Autodesk Fusion 360 part; units mm, degrees
note: some values were not read from the file. Chosen so that the rebuilt part matches the saved one: which face or edge a step refers to. Set by a fixed rule: which sketch regions a step uses.
(part 3 of 3)
sketch "Hex Side" plane through (0, 0, 0) normal (1, 0, 0) x (0, 1, 0)
  line L0 (0, 0) -> (-0.001, 0) construction
  line L1 (-0.001, 0) -> (-0.001, 1) construction
  line L2 (-0.001, 1) -> (0, 1) construction
  line L3 (0, 1) -> (0, 0) construction
  line L4 (-1.9518, 4.3789) -> (-3.9026, 1)
  line L5 (-3.9026, 1) -> (-1.9518, -2.3789)
  line L6 (-1.9518, -2.3789) -> (1.9498, -2.3789)
  line L7 (1.9498, -2.3789) -> (3.9006, 1)
  line L8 (3.9006, 1) -> (1.9498, 4.3789)
  line L9 (1.9498, 4.3789) -> (-1.9518, 4.3789)
  line L10 (-0.001, 1) -> (2.9252, 2.6894) construction
  line L11 (-0.001, 1) -> (-0.001, -2.3789) construction
  line L12 (4.9396, 8.3576) -> (2.9888, 4.9787)
  line L13 (8.8412, 8.3576) -> (4.9396, 8.3576)
  line L14 (2.9888, 4.9787) -> (4.9396, 1.5999)
  line L15 (4.9396, 1.5999) -> (8.8412, 1.5999)
  line L16 (8.8412, 1.5999) -> (10.792, 4.9787)
  line L17 (10.792, 4.9787) -> (8.8412, 8.3576)
  line L18 (2.9252, 2.6894) -> (3.9644, 3.2894)
  line L19 (-61.6828, -7.5574) -> (-65.5844, -7.5574)
  line L20 (-65.5844, -7.5574) -> (-67.5352, -10.9363)
  line L21 (-59.732, -10.9363) -> (-61.6828, -7.5574)
  line L22 (-61.6828, -14.3151) -> (-59.732, -10.9363)
  line L23 (-65.5844, -14.3151) -> (-61.6828, -14.3151)
  line L24 (-67.5352, -10.9363) -> (-65.5844, -14.3151)
  line L25 (-66.6234, -14.915) -> (-68.5742, -11.5361)
  line L26 (-68.5742, -18.2939) -> (-66.6234, -14.915)
  line L27 (-72.4758, -18.2939) -> (-68.5742, -18.2939)
  line L28 (-68.5742, -11.5361) -> (-72.4758, -11.5361)
  line L29 (-72.4758, -11.5361) -> (-74.4266, -14.915)
  line L30 (-74.4266, -14.915) -> (-72.4758, -18.2939)
  line L31 (-47.578, 0.4001) -> (-51.4796, 0.4001)
  line L32 (-51.4796, 0.4001) -> (-53.4304, -2.9788)
  line L33 (-45.6272, -2.9788) -> (-47.578, 0.4001)
  line L34 (-47.578, -6.3576) -> (-45.6272, -2.9788)
  line L35 (-51.4796, -6.3576) -> (-47.578, -6.3576)
  line L36 (-53.4304, -2.9788) -> (-51.4796, -6.3576)
  line L37 (-52.5186, -6.9575) -> (-54.4694, -3.5786)
  line L38 (-54.4694, -10.3364) -> (-52.5186, -6.9575)
  line L39 (-58.371, -10.3364) -> (-54.4694, -10.3364)
  line L40 (-54.4694, -3.5786) -> (-58.371, -3.5786)
  line L41 (-58.371, -3.5786) -> (-60.3218, -6.9575)
  line L42 (-60.3218, -6.9575) -> (-58.371, -10.3364)
  line L43 (-0.001, 4.3789) -> (-0.001, 5.5789)
  line L44 (3.9006, 1) -> (9.0022, 1) construction
  line L45 (9.0022, 1) -> (9.0022, -0.4851) construction
  line L46 (-47.578, -7.5574) -> (-51.4796, -7.5574)
  line L47 (-51.4796, -7.5574) -> (-53.4304, -10.9363)
  line L48 (-45.6272, -10.9363) -> (-47.578, -7.5574)
  line L49 (-47.578, -14.3151) -> (-45.6272, -10.9363)
  line L50 (-51.4796, -14.3151) -> (-47.578, -14.3151)
  line L51 (-53.4304, -10.9363) -> (-51.4796, -14.3151)
  line L52 (-52.5186, -14.915) -> (-54.4694, -11.5361)
  line L53 (-54.4694, -18.2939) -> (-52.5186, -14.915)
  line L54 (-58.371, -18.2939) -> (-54.4694, -18.2939)
  line L55 (-54.4694, -11.5361) -> (-58.371, -11.5361)
  line L56 (-58.371, -11.5361) -> (-60.3218, -14.915)
  line L57 (-60.3218, -14.915) -> (-58.371, -18.2939)
  line L58 (-61.6828, 0.4001) -> (-65.5844, 0.4001)
  line L59 (-65.5844, 0.4001) -> (-67.5352, -2.9788)
  line L60 (-59.732, -2.9788) -> (-61.6828, 0.4001)
  line L61 (-61.6828, -6.3576) -> (-59.732, -2.9788)
  line L62 (-65.5844, -6.3576) -> (-61.6828, -6.3576)
  line L63 (-67.5352, -2.9788) -> (-65.5844, -6.3576)
  line L64 (-66.6234, -6.9575) -> (-68.5742, -3.5786)
  line L65 (-68.5742, -10.3364) -> (-66.6234, -6.9575)
  line L66 (-72.4758, -10.3364) -> (-68.5742, -10.3364)
  line L67 (-68.5742, -3.5786) -> (-72.4758, -3.5786)
  line L68 (-72.4758, -3.5786) -> (-74.4266, -6.9575)
  line L69 (-74.4266, -6.9575) -> (-72.4758, -10.3364)
  line L70 (-61.6828, 8.3576) -> (-65.5844, 8.3576)
  line L71 (-65.5844, 8.3576) -> (-67.5352, 4.9787)
  line L72 (-59.732, 4.9787) -> (-61.6828, 8.3576)
  line L73 (-61.6828, 1.5999) -> (-59.732, 4.9787)
  line L74 (-65.5844, 1.5999) -> (-61.6828, 1.5999)
  line L75 (-67.5352, 4.9787) -> (-65.5844, 1.5999)
  line L76 (-66.6234, 1) -> (-68.5742, 4.3789)
  line L77 (-68.5742, -2.3789) -> (-66.6234, 1)
  line L78 (-72.4758, -2.3789) -> (-68.5742, -2.3789)
  line L79 (-68.5742, 4.3789) -> (-72.4758, 4.3789)
  line L80 (-72.4758, 4.3789) -> (-74.4266, 1)
  line L81 (-74.4266, 1) -> (-72.4758, -2.3789)
  line L82 (9.0022, 1) -> (10.2022, 1) construction
  line L83 (-33.4732, -7.5574) -> (-37.3748, -7.5574)
  line L84 (-37.3748, -7.5574) -> (-39.3256, -10.9363)
  line L85 (-31.5224, -10.9363) -> (-33.4732, -7.5574)
  line L86 (-33.4732, -14.3151) -> (-31.5224, -10.9363)
  line L87 (-37.3748, -14.3151) -> (-33.4732, -14.3151)
  line L88 (-39.3256, -10.9363) -> (-37.3748, -14.3151)
  line L89 (-38.4138, -14.915) -> (-40.3646, -11.5361)
  line L90 (-40.3646, -18.2939) -> (-38.4138, -14.915)
  line L91 (-44.2662, -18.2939) -> (-40.3646, -18.2939)
  line L92 (-40.3646, -11.5361) -> (-44.2662, -11.5361)
  line L93 (-44.2662, -11.5361) -> (-46.217, -14.915)
  line L94 (-46.217, -14.915) -> (-44.2662, -18.2939)
  line L95 (-19.3684, -7.5574) -> (-23.27, -7.5574)
  line L96 (-23.27, -7.5574) -> (-25.2208, -10.9363)
  line L97 (-17.4176, -10.9363) -> (-19.3684, -7.5574)
  line L98 (-19.3684, -14.3151) -> (-17.4176, -10.9363)
  line L99 (-23.27, -14.3151) -> (-19.3684, -14.3151)
  line L100 (-25.2208, -10.9363) -> (-23.27, -14.3151)
  line L101 (-24.309, -14.915) -> (-26.2598, -11.5361)
  line L102 (-26.2598, -18.2939) -> (-24.309, -14.915)
  line L103 (-30.1614, -18.2939) -> (-26.2598, -18.2939)
  line L104 (-26.2598, -11.5361) -> (-30.1614, -11.5361)
  line L105 (-30.1614, -11.5361) -> (-32.1122, -14.915)
  line L106 (-32.1122, -14.915) -> (-30.1614, -18.2939)
  line L107 (-5.2636, -7.5574) -> (-9.1652, -7.5574)
  line L108 (-9.1652, -7.5574) -> (-11.116, -10.9363)
  line L109 (-3.3128, -10.9363) -> (-5.2636, -7.5574)
  line L110 (-5.2636, -14.3151) -> (-3.3128, -10.9363)
  line L111 (-9.1652, -14.3151) -> (-5.2636, -14.3151)
  line L112 (-11.116, -10.9363) -> (-9.1652, -14.3151)
  line L113 (-10.2042, -14.915) -> (-12.155, -11.5361)
  line L114 (-12.155, -18.2939) -> (-10.2042, -14.915)
  line L115 (-16.0566, -18.2939) -> (-12.155, -18.2939)
  line L116 (-12.155, -11.5361) -> (-16.0566, -11.5361)
  line L117 (-16.0566, -11.5361) -> (-18.0074, -14.915)
  line L118 (-18.0074, -14.915) -> (-16.0566, -18.2939)
  line L119 (8.8412, -7.5574) -> (4.9396, -7.5574)
  line L120 (4.9396, -7.5574) -> (2.9888, -10.9363)
  line L121 (10.792, -10.9363) -> (8.8412, -7.5574)
  line L122 (8.8412, -14.3151) -> (10.792, -10.9363)
  line L123 (4.9396, -14.3151) -> (8.8412, -14.3151)
  line L124 (2.9888, -10.9363) -> (4.9396, -14.3151)
  line L125 (3.9006, -14.915) -> (1.9498, -11.5361)
  line L126 (1.9498, -18.2939) -> (3.9006, -14.915)
  line L127 (-1.9518, -18.2939) -> (1.9498, -18.2939)
  line L128 (1.9498, -11.5361) -> (-1.9518, -11.5361)
  line L129 (-1.9518, -11.5361) -> (-3.9026, -14.915)
  line L130 (-3.9026, -14.915) -> (-1.9518, -18.2939)
  line L131 (22.946, -7.5574) -> (19.0444, -7.5574)
  line L132 (19.0444, -7.5574) -> (17.0936, -10.9363)
  line L133 (24.8968, -10.9363) -> (22.946, -7.5574)
  line L134 (22.946, -14.3151) -> (24.8968, -10.9363)
  line L135 (19.0444, -14.3151) -> (22.946, -14.3151)
  line L136 (17.0936, -10.9363) -> (19.0444, -14.3151)
  line L137 (18.0054, -14.915) -> (16.0546, -11.5361)
  line L138 (16.0546, -18.2939) -> (18.0054, -14.915)
  line L139 (12.153, -18.2939) -> (16.0546, -18.2939)
  line L140 (16.0546, -11.5361) -> (12.153, -11.5361)
  line L141 (12.153, -11.5361) -> (10.2022, -14.915)
  line L142 (10.2022, -14.915) -> (12.153, -18.2939)
  line L143 (37.0508, -7.5574) -> (33.1492, -7.5574)
  line L144 (33.1492, -7.5574) -> (31.1984, -10.9363)
  line L145 (39.0016, -10.9363) -> (37.0508, -7.5574)
  line L146 (37.0508, -14.3151) -> (39.0016, -10.9363)
  line L147 (33.1492, -14.3151) -> (37.0508, -14.3151)
  line L148 (31.1984, -10.9363) -> (33.1492, -14.3151)
  line L149 (32.1102, -14.915) -> (30.1594, -11.5361)
  line L150 (30.1594, -18.2939) -> (32.1102, -14.915)
  line L151 (26.2578, -18.2939) -> (30.1594, -18.2939)
  line L152 (30.1594, -11.5361) -> (26.2578, -11.5361)
  line L153 (26.2578, -11.5361) -> (24.307, -14.915)
  line L154 (24.307, -14.915) -> (26.2578, -18.2939)
  line L155 (51.1556, -7.5574) -> (47.254, -7.5574)
  line L156 (47.254, -7.5574) -> (45.3032, -10.9363)
  line L157 (53.1064, -10.9363) -> (51.1556, -7.5574)
  line L158 (51.1556, -14.3151) -> (53.1064, -10.9363)
  line L159 (47.254, -14.3151) -> (51.1556, -14.3151)
  line L160 (45.3032, -10.9363) -> (47.254, -14.3151)
  line L161 (46.215, -14.915) -> (44.2642, -11.5361)
  line L162 (44.2642, -18.2939) -> (46.215, -14.915)
  line L163 (40.3626, -18.2939) -> (44.2642, -18.2939)
  line L164 (44.2642, -11.5361) -> (40.3626, -11.5361)
  line L165 (40.3626, -11.5361) -> (38.4118, -14.915)
  line L166 (38.4118, -14.915) -> (40.3626, -18.2939)
  line L167 (65.2604, -7.5574) -> (61.3588, -7.5574)
  line L168 (61.3588, -7.5574) -> (59.408, -10.9363)
  line L169 (67.2112, -10.9363) -> (65.2604, -7.5574)
  line L170 (65.2604, -14.3151) -> (67.2112, -10.9363)
  line L171 (61.3588, -14.3151) -> (65.2604, -14.3151)
  line L172 (59.408, -10.9363) -> (61.3588, -14.3151)
  line L173 (60.3198, -14.915) -> (58.369, -11.5361)
  line L174 (58.369, -18.2939) -> (60.3198, -14.915)
  line L175 (54.4674, -18.2939) -> (58.369, -18.2939)
  line L176 (58.369, -11.5361) -> (54.4674, -11.5361)
  line L177 (54.4674, -11.5361) -> (52.5166, -14.915)
  line L178 (52.5166, -14.915) -> (54.4674, -18.2939)
  line L179 (79.3652, -7.5574) -> (75.4636, -7.5574)
  line L180 (75.4636, -7.5574) -> (73.5128, -10.9363)
  line L181 (81.316, -10.9363) -> (79.3652, -7.5574)
  line L182 (79.3652, -14.3151) -> (81.316, -10.9363)
  line L183 (75.4636, -14.3151) -> (79.3652, -14.3151)
  line L184 (73.5128, -10.9363) -> (75.4636, -14.3151)
  line L185 (74.4246, -14.915) -> (72.4738, -11.5361)
  line L186 (72.4738, -18.2939) -> (74.4246, -14.915)
  line L187 (68.5722, -18.2939) -> (72.4738, -18.2939)
  line L188 (72.4738, -11.5361) -> (68.5722, -11.5361)
  line L189 (68.5722, -11.5361) -> (66.6214, -14.915)
  line L190 (66.6214, -14.915) -> (68.5722, -18.2939)
  line L191 (-33.4732, 0.4001) -> (-37.3748, 0.4001)
  line L192 (-37.3748, 0.4001) -> (-39.3256, -2.9788)
  line L193 (-31.5224, -2.9788) -> (-33.4732, 0.4001)
  line L194 (-33.4732, -6.3576) -> (-31.5224, -2.9788)
  line L195 (-37.3748, -6.3576) -> (-33.4732, -6.3576)
  line L196 (-39.3256, -2.9788) -> (-37.3748, -6.3576)
  line L197 (-38.4138, -6.9575) -> (-40.3646, -3.5786)
  line L198 (-40.3646, -10.3364) -> (-38.4138, -6.9575)
  line L199 (-44.2662, -10.3364) -> (-40.3646, -10.3364)
  line L200 (-40.3646, -3.5786) -> (-44.2662, -3.5786)
  line L201 (-44.2662, -3.5786) -> (-46.217, -6.9575)
  line L202 (-46.217, -6.9575) -> (-44.2662, -10.3364)
  line L203 (-19.3684, 0.4001) -> (-23.27, 0.4001)
  line L204 (-23.27, 0.4001) -> (-25.2208, -2.9788)
  line L205 (-17.4176, -2.9788) -> (-19.3684, 0.4001)
  line L206 (-19.3684, -6.3576) -> (-17.4176, -2.9788)
  line L207 (-23.27, -6.3576) -> (-19.3684, -6.3576)
  line L208 (-25.2208, -2.9788) -> (-23.27, -6.3576)
  line L209 (-24.309, -6.9575) -> (-26.2598, -3.5786)
  line L210 (-26.2598, -10.3364) -> (-24.309, -6.9575)
  line L211 (-30.1614, -10.3364) -> (-26.2598, -10.3364)
  line L212 (-26.2598, -3.5786) -> (-30.1614, -3.5786)
  line L213 (-30.1614, -3.5786) -> (-32.1122, -6.9575)
  line L214 (-32.1122, -6.9575) -> (-30.1614, -10.3364)
  line L215 (-5.2636, 0.4001) -> (-9.1652, 0.4001)
  line L216 (-9.1652, 0.4001) -> (-11.116, -2.9788)
  line L217 (-3.3128, -2.9788) -> (-5.2636, 0.4001)
  line L218 (-5.2636, -6.3576) -> (-3.3128, -2.9788)
  line L219 (-9.1652, -6.3576) -> (-5.2636, -6.3576)
  line L220 (-11.116, -2.9788) -> (-9.1652, -6.3576)
  line L221 (-10.2042, -6.9575) -> (-12.155, -3.5786)
  line L222 (-12.155, -10.3364) -> (-10.2042, -6.9575)
  line L223 (-16.0566, -10.3364) -> (-12.155, -10.3364)
  line L224 (-12.155, -3.5786) -> (-16.0566, -3.5786)
  line L225 (-16.0566, -3.5786) -> (-18.0074, -6.9575)
  line L226 (-18.0074, -6.9575) -> (-16.0566, -10.3364)
  line L227 (8.8412, 0.4001) -> (4.9396, 0.4001)
  line L228 (4.9396, 0.4001) -> (2.9888, -2.9788)
  line L229 (10.792, -2.9788) -> (8.8412, 0.4001)
  line L230 (8.8412, -6.3576) -> (10.792, -2.9788)
  line L231 (4.9396, -6.3576) -> (8.8412, -6.3576)
  line L232 (2.9888, -2.9788) -> (4.9396, -6.3576)
  line L233 (3.9006, -6.9575) -> (1.9498, -3.5786)
  line L234 (1.9498, -10.3364) -> (3.9006, -6.9575)
  line L235 (-1.9518, -10.3364) -> (1.9498, -10.3364)
  line L236 (1.9498, -3.5786) -> (-1.9518, -3.5786)
  line L237 (-1.9518, -3.5786) -> (-3.9026, -6.9575)
  line L238 (-3.9026, -6.9575) -> (-1.9518, -10.3364)
  line L239 (22.946, 0.4001) -> (19.0444, 0.4001)
  line L240 (19.0444, 0.4001) -> (17.0936, -2.9788)
  line L241 (24.8968, -2.9788) -> (22.946, 0.4001)
  line L242 (22.946, -6.3576) -> (24.8968, -2.9788)
  line L243 (19.0444, -6.3576) -> (22.946, -6.3576)
  line L244 (17.0936, -2.9788) -> (19.0444, -6.3576)
  line L245 (18.0054, -6.9575) -> (16.0546, -3.5786)
  line L246 (16.0546, -10.3364) -> (18.0054, -6.9575)
  line L247 (12.153, -10.3364) -> (16.0546, -10.3364)
  line L248 (16.0546, -3.5786) -> (12.153, -3.5786)
  line L249 (12.153, -3.5786) -> (10.2022, -6.9575)
  line L250 (10.2022, -6.9575) -> (12.153, -10.3364)
  line L251 (37.0508, 0.4001) -> (33.1492, 0.4001)
  line L252 (33.1492, 0.4001) -> (31.1984, -2.9788)
  line L253 (39.0016, -2.9788) -> (37.0508, 0.4001)
  line L254 (37.0508, -6.3576) -> (39.0016, -2.9788)
  line L255 (33.1492, -6.3576) -> (37.0508, -6.3576)
  line L256 (31.1984, -2.9788) -> (33.1492, -6.3576)
  line L257 (32.1102, -6.9575) -> (30.1594, -3.5786)
  line L258 (30.1594, -10.3364) -> (32.1102, -6.9575)
  line L259 (26.2578, -10.3364) -> (30.1594, -10.3364)
  line L260 (30.1594, -3.5786) -> (26.2578, -3.5786)
  line L261 (26.2578, -3.5786) -> (24.307, -6.9575)
  line L262 (24.307, -6.9575) -> (26.2578, -10.3364)
  line L263 (51.1556, 0.4001) -> (47.254, 0.4001)
  line L264 (47.254, 0.4001) -> (45.3032, -2.9788)
  line L265 (53.1064, -2.9788) -> (51.1556, 0.4001)
  line L266 (51.1556, -6.3576) -> (53.1064, -2.9788)
  line L267 (47.254, -6.3576) -> (51.1556, -6.3576)
  line L268 (45.3032, -2.9788) -> (47.254, -6.3576)
  line L269 (46.215, -6.9575) -> (44.2642, -3.5786)
  line L270 (44.2642, -10.3364) -> (46.215, -6.9575)
  line L271 (40.3626, -10.3364) -> (44.2642, -10.3364)
  line L272 (44.2642, -3.5786) -> (40.3626, -3.5786)
  line L273 (40.3626, -3.5786) -> (38.4118, -6.9575)
  line L274 (38.4118, -6.9575) -> (40.3626, -10.3364)
  line L275 (65.2604, 0.4001) -> (61.3588, 0.4001)
  line L276 (61.3588, 0.4001) -> (59.408, -2.9788)
  line L277 (67.2112, -2.9788) -> (65.2604, 0.4001)
  line L278 (65.2604, -6.3576) -> (67.2112, -2.9788)
  line L279 (61.3588, -6.3576) -> (65.2604, -6.3576)
  line L280 (59.408, -2.9788) -> (61.3588, -6.3576)
  line L281 (60.3198, -6.9575) -> (58.369, -3.5786)
  line L282 (58.369, -10.3364) -> (60.3198, -6.9575)
  line L283 (54.4674, -10.3364) -> (58.369, -10.3364)
  line L284 (58.369, -3.5786) -> (54.4674, -3.5786)
  line L285 (54.4674, -3.5786) -> (52.5166, -6.9575)
  line L286 (52.5166, -6.9575) -> (54.4674, -10.3364)
  line L287 (79.3652, 0.4001) -> (75.4636, 0.4001)
  line L288 (75.4636, 0.4001) -> (73.5128, -2.9788)
  line L289 (81.316, -2.9788) -> (79.3652, 0.4001)
  line L290 (79.3652, -6.3576) -> (81.316, -2.9788)
  line L291 (75.4636, -6.3576) -> (79.3652, -6.3576)
  line L292 (73.5128, -2.9788) -> (75.4636, -6.3576)
  line L293 (74.4246, -6.9575) -> (72.4738, -3.5786)
  line L294 (72.4738, -10.3364) -> (74.4246, -6.9575)
  line L295 (68.5722, -10.3364) -> (72.4738, -10.3364)
  line L296 (72.4738, -3.5786) -> (68.5722, -3.5786)
  line L297 (68.5722, -3.5786) -> (66.6214, -6.9575)
  line L298 (66.6214, -6.9575) -> (68.5722, -10.3364)
  line L299 (-47.578, 8.3576) -> (-51.4796, 8.3576)
  line L300 (-51.4796, 8.3576) -> (-53.4304, 4.9787)
  line L301 (-45.6272, 4.9787) -> (-47.578, 8.3576)
  line L302 (-47.578, 1.5999) -> (-45.6272, 4.9787)
  line L303 (-51.4796, 1.5999) -> (-47.578, 1.5999)
  line L304 (-53.4304, 4.9787) -> (-51.4796, 1.5999)
  line L305 (-52.5186, 1) -> (-54.4694, 4.3789)
  line L306 (-54.4694, -2.3789) -> (-52.5186, 1)
  line L307 (-58.371, -2.3789) -> (-54.4694, -2.3789)
  line L308 (-54.4694, 4.3789) -> (-58.371, 4.3789)
  line L309 (-58.371, 4.3789) -> (-60.3218, 1)
  line L310 (-60.3218, 1) -> (-58.371, -2.3789)
  line L311 (-33.4732, 8.3576) -> (-37.3748, 8.3576)
  line L312 (-37.3748, 8.3576) -> (-39.3256, 4.9787)
  line L313 (-31.5224, 4.9787) -> (-33.4732, 8.3576)
  line L314 (-33.4732, 1.5999) -> (-31.5224, 4.9787)
  line L315 (-37.3748, 1.5999) -> (-33.4732, 1.5999)
  line L316 (-39.3256, 4.9787) -> (-37.3748, 1.5999)
  line L317 (-38.4138, 1) -> (-40.3646, 4.3789)
  line L318 (-40.3646, -2.3789) -> (-38.4138, 1)
  line L319 (-44.2662, -2.3789) -> (-40.3646, -2.3789)
  line L320 (-40.3646, 4.3789) -> (-44.2662, 4.3789)
  line L321 (-44.2662, 4.3789) -> (-46.217, 1)
  line L322 (-46.217, 1) -> (-44.2662, -2.3789)
  line L323 (-19.3684, 8.3576) -> (-23.27, 8.3576)
  line L324 (-23.27, 8.3576) -> (-25.2208, 4.9787)
  line L325 (-17.4176, 4.9787) -> (-19.3684, 8.3576)
  line L326 (-19.3684, 1.5999) -> (-17.4176, 4.9787)
  line L327 (-23.27, 1.5999) -> (-19.3684, 1.5999)
  line L328 (-25.2208, 4.9787) -> (-23.27, 1.5999)
  line L329 (-24.309, 1) -> (-26.2598, 4.3789)
  line L330 (-26.2598, -2.3789) -> (-24.309, 1)
  line L331 (-30.1614, -2.3789) -> (-26.2598, -2.3789)
  line L332 (-26.2598, 4.3789) -> (-30.1614, 4.3789)
  line L333 (-30.1614, 4.3789) -> (-32.1122, 1)
  line L334 (-32.1122, 1) -> (-30.1614, -2.3789)
  line L335 (-5.2636, 8.3576) -> (-9.1652, 8.3576)
  line L336 (-9.1652, 8.3576) -> (-11.116, 4.9787)
  line L337 (-3.3128, 4.9787) -> (-5.2636, 8.3576)
  line L338 (-5.2636, 1.5999) -> (-3.3128, 4.9787)
  line L339 (-9.1652, 1.5999) -> (-5.2636, 1.5999)
  line L340 (-11.116, 4.9787) -> (-9.1652, 1.5999)
  line L341 (-10.2042, 1) -> (-12.155, 4.3789)
  line L342 (-12.155, -2.3789) -> (-10.2042, 1)
  line L343 (-16.0566, -2.3789) -> (-12.155, -2.3789)
  line L344 (-12.155, 4.3789) -> (-16.0566, 4.3789)
  line L345 (-16.0566, 4.3789) -> (-18.0074, 1)
  line L346 (-18.0074, 1) -> (-16.0566, -2.3789)
  line L347 (22.946, 8.3576) -> (19.0444, 8.3576)
  line L348 (19.0444, 8.3576) -> (17.0936, 4.9787)
  line L349 (24.8968, 4.9787) -> (22.946, 8.3576)
  line L350 (22.946, 1.5999) -> (24.8968, 4.9787)
  line L351 (19.0444, 1.5999) -> (22.946, 1.5999)
  line L352 (17.0936, 4.9787) -> (19.0444, 1.5999)
  line L353 (18.0054, 1) -> (16.0546, 4.3789)
  line L354 (16.0546, -2.3789) -> (18.0054, 1)
  line L355 (12.153, -2.3789) -> (16.0546, -2.3789)
  line L356 (16.0546, 4.3789) -> (12.153, 4.3789)
  line L357 (12.153, 4.3789) -> (10.2022, 1)
  line L358 (10.2022, 1) -> (12.153, -2.3789)
  line L359 (37.0508, 8.3576) -> (33.1492, 8.3576)
  line L360 (33.1492, 8.3576) -> (31.1984, 4.9787)
  line L361 (39.0016, 4.9787) -> (37.0508, 8.3576)
  line L362 (37.0508, 1.5999) -> (39.0016, 4.9787)
  line L363 (33.1492, 1.5999) -> (37.0508, 1.5999)
  line L364 (31.1984, 4.9787) -> (33.1492, 1.5999)
  line L365 (32.1102, 1) -> (30.1594, 4.3789)
  line L366 (30.1594, -2.3789) -> (32.1102, 1)
  line L367 (26.2578, -2.3789) -> (30.1594, -2.3789)
  line L368 (30.1594, 4.3789) -> (26.2578, 4.3789)
  line L369 (26.2578, 4.3789) -> (24.307, 1)
  line L370 (24.307, 1) -> (26.2578, -2.3789)
  line L371 (51.1556, 8.3576) -> (47.254, 8.3576)
  line L372 (47.254, 8.3576) -> (45.3032, 4.9787)
  line L373 (53.1064, 4.9787) -> (51.1556, 8.3576)
  line L374 (51.1556, 1.5999) -> (53.1064, 4.9787)
  line L375 (47.254, 1.5999) -> (51.1556, 1.5999)
  line L376 (45.3032, 4.9787) -> (47.254, 1.5999)
  line L377 (46.215, 1) -> (44.2642, 4.3789)
  line L378 (44.2642, -2.3789) -> (46.215, 1)
  line L379 (40.3626, -2.3789) -> (44.2642, -2.3789)
  line L380 (44.2642, 4.3789) -> (40.3626, 4.3789)
  line L381 (40.3626, 4.3789) -> (38.4118, 1)
  line L382 (38.4118, 1) -> (40.3626, -2.3789)
  line L383 (65.2604, 8.3576) -> (61.3588, 8.3576)
  line L384 (61.3588, 8.3576) -> (59.408, 4.9787)
  line L385 (67.2112, 4.9787) -> (65.2604, 8.3576)
  line L386 (65.2604, 1.5999) -> (67.2112, 4.9787)
  line L387 (61.3588, 1.5999) -> (65.2604, 1.5999)
  line L388 (59.408, 4.9787) -> (61.3588, 1.5999)
  line L389 (60.3198, 1) -> (58.369, 4.3789)
  line L390 (58.369, -2.3789) -> (60.3198, 1)
  line L391 (54.4674, -2.3789) -> (58.369, -2.3789)
  line L392 (58.369, 4.3789) -> (54.4674, 4.3789)
  line L393 (54.4674, 4.3789) -> (52.5166, 1)
  line L394 (52.5166, 1) -> (54.4674, -2.3789)
  line L395 (79.3652, 8.3576) -> (75.4636, 8.3576)
  line L396 (75.4636, 8.3576) -> (73.5128, 4.9787)
  line L397 (81.316, 4.9787) -> (79.3652, 8.3576)
  line L398 (79.3652, 1.5999) -> (81.316, 4.9787)
  line L399 (75.4636, 1.5999) -> (79.3652, 1.5999)
  line L400 (73.5128, 4.9787) -> (75.4636, 1.5999)
  line L401 (74.4246, 1) -> (72.4738, 4.3789)
  line L402 (72.4738, -2.3789) -> (74.4246, 1)
  line L403 (68.5722, -2.3789) -> (72.4738, -2.3789)
  line L404 (72.4738, 4.3789) -> (68.5722, 4.3789)
  line L405 (68.5722, 4.3789) -> (66.6214, 1)
  line L406 (66.6214, 1) -> (68.5722, -2.3789)
  line L407 (-61.6828, 16.3151) -> (-65.5844, 16.3151)
  line L408 (-65.5844, 16.3151) -> (-67.5352, 12.9362)
  line L409 (-59.732, 12.9362) -> (-61.6828, 16.3151)
  line L410 (-61.6828, 9.5574) -> (-59.732, 12.9362)
  line L411 (-65.5844, 9.5574) -> (-61.6828, 9.5574)
  line L412 (-67.5352, 12.9362) -> (-65.5844, 9.5574)
  line L413 (-66.6234, 8.9575) -> (-68.5742, 12.3364)
  line L414 (-68.5742, 5.5786) -> (-66.6234, 8.9575)
  line L415 (-72.4758, 5.5786) -> (-68.5742, 5.5786)
  line L416 (-68.5742, 12.3364) -> (-72.4758, 12.3364)
  line L417 (-72.4758, 12.3364) -> (-74.4266, 8.9575)
  line L418 (-74.4266, 8.9575) -> (-72.4758, 5.5786)
  line L419 (-47.578, 16.3151) -> (-51.4796, 16.3151)
  line L420 (-51.4796, 16.3151) -> (-53.4304, 12.9362)
  line L421 (-45.6272, 12.9362) -> (-47.578, 16.3151)
  line L422 (-47.578, 9.5574) -> (-45.6272, 12.9362)
  line L423 (-51.4796, 9.5574) -> (-47.578, 9.5574)
  line L424 (-53.4304, 12.9362) -> (-51.4796, 9.5574)
  line L425 (-52.5186, 8.9575) -> (-54.4694, 12.3364)
  line L426 (-54.4694, 5.5786) -> (-52.5186, 8.9575)
  line L427 (-58.371, 5.5786) -> (-54.4694, 5.5786)
  line L428 (-54.4694, 12.3364) -> (-58.371, 12.3364)
  line L429 (-58.371, 12.3364) -> (-60.3218, 8.9575)
  line L430 (-60.3218, 8.9575) -> (-58.371, 5.5786)
  line L431 (-33.4732, 16.3151) -> (-37.3748, 16.3151)
  line L432 (-37.3748, 16.3151) -> (-39.3256, 12.9362)
  line L433 (-31.5224, 12.9362) -> (-33.4732, 16.3151)
  line L434 (-33.4732, 9.5574) -> (-31.5224, 12.9362)
  line L435 (-37.3748, 9.5574) -> (-33.4732, 9.5574)
  line L436 (-39.3256, 12.9362) -> (-37.3748, 9.5574)
  line L437 (-38.4138, 8.9575) -> (-40.3646, 12.3364)
  line L438 (-40.3646, 5.5786) -> (-38.4138, 8.9575)
  line L439 (-44.2662, 5.5786) -> (-40.3646, 5.5786)
  line L440 (-40.3646, 12.3364) -> (-44.2662, 12.3364)
  line L441 (-44.2662, 12.3364) -> (-46.217, 8.9575)
  line L442 (-46.217, 8.9575) -> (-44.2662, 5.5786)
  line L443 (-19.3684, 16.3151) -> (-23.27, 16.3151)
  line L444 (-23.27, 16.3151) -> (-25.2208, 12.9362)
  line L445 (-17.4176, 12.9362) -> (-19.3684, 16.3151)
  line L446 (-19.3684, 9.5574) -> (-17.4176, 12.9362)
  line L447 (-23.27, 9.5574) -> (-19.3684, 9.5574)
  line L448 (-25.2208, 12.9362) -> (-23.27, 9.5574)
  line L449 (-24.309, 8.9575) -> (-26.2598, 12.3364)
  line L450 (-26.2598, 5.5786) -> (-24.309, 8.9575)
  line L451 (-30.1614, 5.5786) -> (-26.2598, 5.5786)
  line L452 (-26.2598, 12.3364) -> (-30.1614, 12.3364)
  line L453 (-30.1614, 12.3364) -> (-32.1122, 8.9575)
  line L454 (-32.1122, 8.9575) -> (-30.1614, 5.5786)
  line L455 (-5.2636, 16.3151) -> (-9.1652, 16.3151)
  line L456 (-9.1652, 16.3151) -> (-11.116, 12.9362)
  line L457 (-3.3128, 12.9362) -> (-5.2636, 16.3151)
  line L458 (-5.2636, 9.5574) -> (-3.3128, 12.9362)
  line L459 (-9.1652, 9.5574) -> (-5.2636, 9.5574)
  line L460 (-11.116, 12.9362) -> (-9.1652, 9.5574)
  line L461 (-10.2042, 8.9575) -> (-12.155, 12.3364)
  line L462 (-12.155, 5.5786) -> (-10.2042, 8.9575)
  line L463 (-16.0566, 5.5786) -> (-12.155, 5.5786)
  line L464 (-12.155, 12.3364) -> (-16.0566, 12.3364)
  line L465 (-16.0566, 12.3364) -> (-18.0074, 8.9575)
  line L466 (-18.0074, 8.9575) -> (-16.0566, 5.5786)
  line L467 (8.8412, 16.3151) -> (4.9396, 16.3151)
  line L468 (4.9396, 16.3151) -> (2.9888, 12.9362)
  line L469 (10.792, 12.9362) -> (8.8412, 16.3151)
  line L470 (8.8412, 9.5574) -> (10.792, 12.9362)
  line L471 (4.9396, 9.5574) -> (8.8412, 9.5574)
  line L472 (2.9888, 12.9362) -> (4.9396, 9.5574)
  line L473 (3.9006, 8.9575) -> (1.9498, 12.3364)
  line L474 (1.9498, 5.5786) -> (3.9006, 8.9575)
  line L475 (-1.9518, 5.5786) -> (1.9498, 5.5786)
  line L476 (1.9498, 12.3364) -> (-1.9518, 12.3364)
  line L477 (-1.9518, 12.3364) -> (-3.9026, 8.9575)
  line L478 (-3.9026, 8.9575) -> (-1.9518, 5.5786)
  line L479 (22.946, 16.3151) -> (19.0444, 16.3151)
  line L480 (19.0444, 16.3151) -> (17.0936, 12.9362)
  line L481 (24.8968, 12.9362) -> (22.946, 16.3151)
  line L482 (22.946, 9.5574) -> (24.8968, 12.9362)
  line L483 (19.0444, 9.5574) -> (22.946, 9.5574)
  line L484 (17.0936, 12.9362) -> (19.0444, 9.5574)
  line L485 (18.0054, 8.9575) -> (16.0546, 12.3364)
  line L486 (16.0546, 5.5786) -> (18.0054, 8.9575)
  line L487 (12.153, 5.5786) -> (16.0546, 5.5786)
  line L488 (16.0546, 12.3364) -> (12.153, 12.3364)
  line L489 (12.153, 12.3364) -> (10.2022, 8.9575)
  line L490 (10.2022, 8.9575) -> (12.153, 5.5786)
  line L491 (37.0508, 16.3151) -> (33.1492, 16.3151)
  line L492 (33.1492, 16.3151) -> (31.1984, 12.9362)
  line L493 (39.0016, 12.9362) -> (37.0508, 16.3151)
  line L494 (37.0508, 9.5574) -> (39.0016, 12.9362)
  line L495 (33.1492, 9.5574) -> (37.0508, 9.5574)
  line L496 (31.1984, 12.9362) -> (33.1492, 9.5574)
  line L497 (32.1102, 8.9575) -> (30.1594, 12.3364)
  line L498 (30.1594, 5.5786) -> (32.1102, 8.9575)
  line L499 (26.2578, 5.5786) -> (30.1594, 5.5786)
  line L500 (30.1594, 12.3364) -> (26.2578, 12.3364)
  line L501 (26.2578, 12.3364) -> (24.307, 8.9575)
  line L502 (24.307, 8.9575) -> (26.2578, 5.5786)
  line L503 (51.1556, 16.3151) -> (47.254, 16.3151)
  line L504 (47.254, 16.3151) -> (45.3032, 12.9362)
  line L505 (53.1064, 12.9362) -> (51.1556, 16.3151)
  line L506 (51.1556, 9.5574) -> (53.1064, 12.9362)
  line L507 (47.254, 9.5574) -> (51.1556, 9.5574)
  line L508 (45.3032, 12.9362) -> (47.254, 9.5574)
  line L509 (46.215, 8.9575) -> (44.2642, 12.3364)
  line L510 (44.2642, 5.5786) -> (46.215, 8.9575)
  line L511 (40.3626, 5.5786) -> (44.2642, 5.5786)
  line L512 (44.2642, 12.3364) -> (40.3626, 12.3364)
  line L513 (40.3626, 12.3364) -> (38.4118, 8.9575)
  line L514 (38.4118, 8.9575) -> (40.3626, 5.5786)
  line L515 (65.2604, 16.3151) -> (61.3588, 16.3151)
  line L516 (61.3588, 16.3151) -> (59.408, 12.9362)
  line L517 (67.2112, 12.9362) -> (65.2604, 16.3151)
  line L518 (65.2604, 9.5574) -> (67.2112, 12.9362)
  line L519 (61.3588, 9.5574) -> (65.2604, 9.5574)
  line L520 (59.408, 12.9362) -> (61.3588, 9.5574)
  line L521 (60.3198, 8.9575) -> (58.369, 12.3364)
  line L522 (58.369, 5.5786) -> (60.3198, 8.9575)
  line L523 (54.4674, 5.5786) -> (58.369, 5.5786)
  line L524 (58.369, 12.3364) -> (54.4674, 12.3364)
  line L525 (54.4674, 12.3364) -> (52.5166, 8.9575)
  line L526 (52.5166, 8.9575) -> (54.4674, 5.5786)
  line L527 (79.3652, 16.3151) -> (75.4636, 16.3151)
  line L528 (75.4636, 16.3151) -> (73.5128, 12.9362)
  line L529 (81.316, 12.9362) -> (79.3652, 16.3151)
  line L530 (79.3652, 9.5574) -> (81.316, 12.9362)
  line L531 (75.4636, 9.5574) -> (79.3652, 9.5574)
  line L532 (73.5128, 12.9362) -> (75.4636, 9.5574)
  line L533 (74.4246, 8.9575) -> (72.4738, 12.3364)
  line L534 (72.4738, 5.5786) -> (74.4246, 8.9575)
  line L535 (68.5722, 5.5786) -> (72.4738, 5.5786)
  line L536 (72.4738, 12.3364) -> (68.5722, 12.3364)
  line L537 (68.5722, 12.3364) -> (66.6214, 8.9575)
  line L538 (66.6214, 8.9575) -> (68.5722, 5.5786)
  line L539 (-61.6828, 24.2726) -> (-65.5844, 24.2726)
  line L540 (-65.5844, 24.2726) -> (-67.5352, 20.8937)
  line L541 (-59.732, 20.8937) -> (-61.6828, 24.2726)
  line L542 (-61.6828, 17.5149) -> (-59.732, 20.8937)
  line L543 (-65.5844, 17.5149) -> (-61.6828, 17.5149)
  line L544 (-67.5352, 20.8937) -> (-65.5844, 17.5149)
  line L545 (-66.6234, 16.915) -> (-68.5742, 20.2939)
  line L546 (-68.5742, 13.5361) -> (-66.6234, 16.915)
  line L547 (-72.4758, 13.5361) -> (-68.5742, 13.5361)
  line L548 (-68.5742, 20.2939) -> (-72.4758, 20.2939)
  line L549 (-72.4758, 20.2939) -> (-74.4266, 16.915)
  line L550 (-74.4266, 16.915) -> (-72.4758, 13.5361)
  line L551 (-47.578, 24.2726) -> (-51.4796, 24.2726)
  line L552 (-51.4796, 24.2726) -> (-53.4304, 20.8937)
  line L553 (-45.6272, 20.8937) -> (-47.578, 24.2726)
  line L554 (-47.578, 17.5149) -> (-45.6272, 20.8937)
  line L555 (-51.4796, 17.5149) -> (-47.578, 17.5149)
  line L556 (-53.4304, 20.8937) -> (-51.4796, 17.5149)
  line L557 (-52.5186, 16.915) -> (-54.4694, 20.2939)
  line L558 (-54.4694, 13.5361) -> (-52.5186, 16.915)
  line L559 (-58.371, 13.5361) -> (-54.4694, 13.5361)
  line L560 (-54.4694, 20.2939) -> (-58.371, 20.2939)
  line L561 (-58.371, 20.2939) -> (-60.3218, 16.915)
  line L562 (-60.3218, 16.915) -> (-58.371, 13.5361)
  line L563 (-33.4732, 24.2726) -> (-37.3748, 24.2726)
  line L564 (-37.3748, 24.2726) -> (-39.3256, 20.8937)
  line L565 (-31.5224, 20.8937) -> (-33.4732, 24.2726)
  line L566 (-33.4732, 17.5149) -> (-31.5224, 20.8937)
  line L567 (-37.3748, 17.5149) -> (-33.4732, 17.5149)
  line L568 (-39.3256, 20.8937) -> (-37.3748, 17.5149)
  line L569 (-38.4138, 16.915) -> (-40.3646, 20.2939)
  line L570 (-40.3646, 13.5361) -> (-38.4138, 16.915)
  line L571 (-44.2662, 13.5361) -> (-40.3646, 13.5361)
  line L572 (-40.3646, 20.2939) -> (-44.2662, 20.2939)
  line L573 (-44.2662, 20.2939) -> (-46.217, 16.915)
  line L574 (-46.217, 16.915) -> (-44.2662, 13.5361)
  line L575 (-19.3684, 24.2726) -> (-23.27, 24.2726)
  line L576 (-23.27, 24.2726) -> (-25.2208, 20.8937)
  line L577 (-17.4176, 20.8937) -> (-19.3684, 24.2726)
  line L578 (-19.3684, 17.5149) -> (-17.4176, 20.8937)
  line L579 (-23.27, 17.5149) -> (-19.3684, 17.5149)
  line L580 (-25.2208, 20.8937) -> (-23.27, 17.5149)
  line L581 (-24.309, 16.915) -> (-26.2598, 20.2939)
  line L582 (-26.2598, 13.5361) -> (-24.309, 16.915)
  line L583 (-30.1614, 13.5361) -> (-26.2598, 13.5361)
  line L584 (-26.2598, 20.2939) -> (-30.1614, 20.2939)
  line L585 (-30.1614, 20.2939) -> (-32.1122, 16.915)
  line L586 (-32.1122, 16.915) -> (-30.1614, 13.5361)
  line L587 (-5.2636, 24.2726) -> (-9.1652, 24.2726)
  line L588 (-9.1652, 24.2726) -> (-11.116, 20.8937)
  line L589 (-3.3128, 20.8937) -> (-5.2636, 24.2726)
  line L590 (-5.2636, 17.5149) -> (-3.3128, 20.8937)
  line L591 (-9.1652, 17.5149) -> (-5.2636, 17.5149)
  line L592 (-11.116, 20.8937) -> (-9.1652, 17.5149)
  line L593 (-10.2042, 16.915) -> (-12.155, 20.2939)
  line L594 (-12.155, 13.5361) -> (-10.2042, 16.915)
  line L595 (-16.0566, 13.5361) -> (-12.155, 13.5361)
  line L596 (-12.155, 20.2939) -> (-16.0566, 20.2939)
  line L597 (-16.0566, 20.2939) -> (-18.0074, 16.915)
  line L598 (-18.0074, 16.915) -> (-16.0566, 13.5361)
  line L599 (8.8412, 24.2726) -> (4.9396, 24.2726)
  line L600 (4.9396, 24.2726) -> (2.9888, 20.8937)
  line L601 (10.792, 20.8937) -> (8.8412, 24.2726)
  line L602 (8.8412, 17.5149) -> (10.792, 20.8937)
  line L603 (4.9396, 17.5149) -> (8.8412, 17.5149)
  line L604 (2.9888, 20.8937) -> (4.9396, 17.5149)
  line L605 (3.9006, 16.915) -> (1.9498, 20.2939)
  line L606 (1.9498, 13.5361) -> (3.9006, 16.915)
  line L607 (-1.9518, 13.5361) -> (1.9498, 13.5361)
  line L608 (1.9498, 20.2939) -> (-1.9518, 20.2939)
  line L609 (-1.9518, 20.2939) -> (-3.9026, 16.915)
  line L610 (-3.9026, 16.915) -> (-1.9518, 13.5361)
  line L611 (22.946, 24.2726) -> (19.0444, 24.2726)
  line L612 (19.0444, 24.2726) -> (17.0936, 20.8937)
  line L613 (24.8968, 20.8937) -> (22.946, 24.2726)
  line L614 (22.946, 17.5149) -> (24.8968, 20.8937)
  line L615 (19.0444, 17.5149) -> (22.946, 17.5149)
  line L616 (17.0936, 20.8937) -> (19.0444, 17.5149)
  line L617 (18.0054, 16.915) -> (16.0546, 20.2939)
  line L618 (16.0546, 13.5361) -> (18.0054, 16.915)
  line L619 (12.153, 13.5361) -> (16.0546, 13.5361)
  line L620 (16.0546, 20.2939) -> (12.153, 20.2939)
  line L621 (12.153, 20.2939) -> (10.2022, 16.915)
  line L622 (10.2022, 16.915) -> (12.153, 13.5361)
  line L623 (37.0508, 24.2726) -> (33.1492, 24.2726)
  line L624 (33.1492, 24.2726) -> (31.1984, 20.8937)
  line L625 (39.0016, 20.8937) -> (37.0508, 24.2726)
  line L626 (37.0508, 17.5149) -> (39.0016, 20.8937)
  line L627 (33.1492, 17.5149) -> (37.0508, 17.5149)
  line L628 (31.1984, 20.8937) -> (33.1492, 17.5149)
  line L629 (32.1102, 16.915) -> (30.1594, 20.2939)
  line L630 (30.1594, 13.5361) -> (32.1102, 16.915)
  line L631 (26.2578, 13.5361) -> (30.1594, 13.5361)
  line L632 (30.1594, 20.2939) -> (26.2578, 20.2939)
  line L633 (26.2578, 20.2939) -> (24.307, 16.915)
  line L634 (24.307, 16.915) -> (26.2578, 13.5361)
  line L635 (51.1556, 24.2726) -> (47.254, 24.2726)
  line L636 (47.254, 24.2726) -> (45.3032, 20.8937)
  line L637 (53.1064, 20.8937) -> (51.1556, 24.2726)
  line L638 (51.1556, 17.5149) -> (53.1064, 20.8937)
  line L639 (47.254, 17.5149) -> (51.1556, 17.5149)
  line L640 (45.3032, 20.8937) -> (47.254, 17.5149)
  line L641 (46.215, 16.915) -> (44.2642, 20.2939)
  line L642 (44.2642, 13.5361) -> (46.215, 16.915)
  line L643 (40.3626, 13.5361) -> (44.2642, 13.5361)
  line L644 (44.2642, 20.2939) -> (40.3626, 20.2939)
  line L645 (40.3626, 20.2939) -> (38.4118, 16.915)
  line L646 (38.4118, 16.915) -> (40.3626, 13.5361)
  line L647 (65.2604, 24.2726) -> (61.3588, 24.2726)
  line L648 (61.3588, 24.2726) -> (59.408, 20.8937)
  line L649 (67.2112, 20.8937) -> (65.2604, 24.2726)
  line L650 (65.2604, 17.5149) -> (67.2112, 20.8937)
  line L651 (61.3588, 17.5149) -> (65.2604, 17.5149)
  line L652 (59.408, 20.8937) -> (61.3588, 17.5149)
  line L653 (60.3198, 16.915) -> (58.369, 20.2939)
  line L654 (58.369, 13.5361) -> (60.3198, 16.915)
  line L655 (54.4674, 13.5361) -> (58.369, 13.5361)
  line L656 (58.369, 20.2939) -> (54.4674, 20.2939)
  line L657 (54.4674, 20.2939) -> (52.5166, 16.915)
  line L658 (52.5166, 16.915) -> (54.4674, 13.5361)
  line L659 (79.3652, 24.2726) -> (75.4636, 24.2726)
  line L660 (75.4636, 24.2726) -> (73.5128, 20.8937)
  line L661 (81.316, 20.8937) -> (79.3652, 24.2726)
  line L662 (79.3652, 17.5149) -> (81.316, 20.8937)
  line L663 (75.4636, 17.5149) -> (79.3652, 17.5149)
  line L664 (73.5128, 20.8937) -> (75.4636, 17.5149)
  line L665 (74.4246, 16.915) -> (72.4738, 20.2939)
  line L666 (72.4738, 13.5361) -> (74.4246, 16.915)
  line L667 (68.5722, 13.5361) -> (72.4738, 13.5361)
  line L668 (72.4738, 20.2939) -> (68.5722, 20.2939)
  line L669 (68.5722, 20.2939) -> (66.6214, 16.915)
  line L670 (66.6214, 16.915) -> (68.5722, 13.5361)
  line L671 (-61.6828, 32.2301) -> (-65.5844, 32.2301)
  line L672 (-65.5844, 32.2301) -> (-67.5352, 28.8512)
  line L673 (-59.732, 28.8512) -> (-61.6828, 32.2301)
  line L674 (-61.6828, 25.4724) -> (-59.732, 28.8512)
  line L675 (-65.5844, 25.4724) -> (-61.6828, 25.4724)
  line L676 (-67.5352, 28.8512) -> (-65.5844, 25.4724)
  line L677 (-66.6234, 24.8725) -> (-68.5742, 28.2514)
  line L678 (-68.5742, 21.4936) -> (-66.6234, 24.8725)
  line L679 (-72.4758, 21.4936) -> (-68.5742, 21.4936)
  line L680 (-68.5742, 28.2514) -> (-72.4758, 28.2514)
  line L681 (-72.4758, 28.2514) -> (-74.4266, 24.8725)
  line L682 (-74.4266, 24.8725) -> (-72.4758, 21.4936)
  line L683 (-47.578, 32.2301) -> (-51.4796, 32.2301)
  line L684 (-51.4796, 32.2301) -> (-53.4304, 28.8512)
  line L685 (-45.6272, 28.8512) -> (-47.578, 32.2301)
  line L686 (-47.578, 25.4724) -> (-45.6272, 28.8512)
  line L687 (-51.4796, 25.4724) -> (-47.578, 25.4724)
  line L688 (-53.4304, 28.8512) -> (-51.4796, 25.4724)
  line L689 (-52.5186, 24.8725) -> (-54.4694, 28.2514)
  line L690 (-54.4694, 21.4936) -> (-52.5186, 24.8725)
  line L691 (-58.371, 21.4936) -> (-54.4694, 21.4936)
  line L692 (-54.4694, 28.2514) -> (-58.371, 28.2514)
  line L693 (-58.371, 28.2514) -> (-60.3218, 24.8725)
  line L694 (-60.3218, 24.8725) -> (-58.371, 21.4936)
  line L695 (-33.4732, 32.2301) -> (-37.3748, 32.2301)
  line L696 (-37.3748, 32.2301) -> (-39.3256, 28.8512)
  line L697 (-31.5224, 28.8512) -> (-33.4732, 32.2301)
  line L698 (-33.4732, 25.4724) -> (-31.5224, 28.8512)
  line L699 (-37.3748, 25.4724) -> (-33.4732, 25.4724)
  line L700 (-39.3256, 28.8512) -> (-37.3748, 25.4724)
  line L701 (-38.4138, 24.8725) -> (-40.3646, 28.2514)
  line L702 (-40.3646, 21.4936) -> (-38.4138, 24.8725)
  line L703 (-44.2662, 21.4936) -> (-40.3646, 21.4936)
  line L704 (-40.3646, 28.2514) -> (-44.2662, 28.2514)
  line L705 (-44.2662, 28.2514) -> (-46.217, 24.8725)
  line L706 (-46.217, 24.8725) -> (-44.2662, 21.4936)
  line L707 (-19.3684, 32.2301) -> (-23.27, 32.2301)
  line L708 (-23.27, 32.2301) -> (-25.2208, 28.8512)
  line L709 (-17.4176, 28.8512) -> (-19.3684, 32.2301)
  line L710 (-19.3684, 25.4724) -> (-17.4176, 28.8512)
  line L711 (-23.27, 25.4724) -> (-19.3684, 25.4724)
  line L712 (-25.2208, 28.8512) -> (-23.27, 25.4724)
  line L713 (-24.309, 24.8725) -> (-26.2598, 28.2514)
  line L714 (-26.2598, 21.4936) -> (-24.309, 24.8725)
  line L715 (-30.1614, 21.4936) -> (-26.2598, 21.4936)
  line L716 (-26.2598, 28.2514) -> (-30.1614, 28.2514)
  line L717 (-30.1614, 28.2514) -> (-32.1122, 24.8725)
  line L718 (-32.1122, 24.8725) -> (-30.1614, 21.4936)
  line L719 (-5.2636, 32.2301) -> (-9.1652, 32.2301)
  line L720 (-9.1652, 32.2301) -> (-11.116, 28.8512)
  line L721 (-3.3128, 28.8512) -> (-5.2636, 32.2301)
  line L722 (-5.2636, 25.4724) -> (-3.3128, 28.8512)
  line L723 (-9.1652, 25.4724) -> (-5.2636, 25.4724)
  line L724 (-11.116, 28.8512) -> (-9.1652, 25.4724)
  line L725 (-10.2042, 24.8725) -> (-12.155, 28.2514)
  line L726 (-12.155, 21.4936) -> (-10.2042, 24.8725)
  line L727 (-16.0566, 21.4936) -> (-12.155, 21.4936)
  line L728 (-12.155, 28.2514) -> (-16.0566, 28.2514)
  line L729 (-16.0566, 28.2514) -> (-18.0074, 24.8725)
  line L730 (-18.0074, 24.8725) -> (-16.0566, 21.4936)
  line L731 (8.8412, 32.2301) -> (4.9396, 32.2301)
  line L732 (4.9396, 32.2301) -> (2.9888, 28.8512)
  line L733 (10.792, 28.8512) -> (8.8412, 32.2301)
  line L734 (8.8412, 25.4724) -> (10.792, 28.8512)
  line L735 (4.9396, 25.4724) -> (8.8412, 25.4724)
  line L736 (2.9888, 28.8512) -> (4.9396, 25.4724)
  line L737 (3.9006, 24.8725) -> (1.9498, 28.2514)
  line L738 (1.9498, 21.4936) -> (3.9006, 24.8725)
  line L739 (-1.9518, 21.4936) -> (1.9498, 21.4936)
  line L740 (1.9498, 28.2514) -> (-1.9518, 28.2514)
  line L741 (-1.9518, 28.2514) -> (-3.9026, 24.8725)
  line L742 (-3.9026, 24.8725) -> (-1.9518, 21.4936)
  line L743 (22.946, 32.2301) -> (19.0444, 32.2301)
  line L744 (19.0444, 32.2301) -> (17.0936, 28.8512)
  line L745 (24.8968, 28.8512) -> (22.946, 32.2301)
  line L746 (22.946, 25.4724) -> (24.8968, 28.8512)
  line L747 (19.0444, 25.4724) -> (22.946, 25.4724)
  line L748 (17.0936, 28.8512) -> (19.0444, 25.4724)
  line L749 (18.0054, 24.8725) -> (16.0546, 28.2514)
  line L750 (16.0546, 21.4936) -> (18.0054, 24.8725)
  line L751 (12.153, 21.4936) -> (16.0546, 21.4936)
  line L752 (16.0546, 28.2514) -> (12.153, 28.2514)
  line L753 (12.153, 28.2514) -> (10.2022, 24.8725)
  line L754 (10.2022, 24.8725) -> (12.153, 21.4936)
  line L755 (37.0508, 32.2301) -> (33.1492, 32.2301)
  line L756 (33.1492, 32.2301) -> (31.1984, 28.8512)
  line L757 (39.0016, 28.8512) -> (37.0508, 32.2301)
  line L758 (37.0508, 25.4724) -> (39.0016, 28.8512)
  line L759 (33.1492, 25.4724) -> (37.0508, 25.4724)
  line L760 (31.1984, 28.8512) -> (33.1492, 25.4724)
  line L761 (32.1102, 24.8725) -> (30.1594, 28.2514)
  line L762 (30.1594, 21.4936) -> (32.1102, 24.8725)
  line L763 (26.2578, 21.4936) -> (30.1594, 21.4936)
  line L764 (30.1594, 28.2514) -> (26.2578, 28.2514)
  line L765 (26.2578, 28.2514) -> (24.307, 24.8725)
  line L766 (24.307, 24.8725) -> (26.2578, 21.4936)
  line L767 (51.1556, 32.2301) -> (47.254, 32.2301)
  line L768 (47.254, 32.2301) -> (45.3032, 28.8512)
  line L769 (53.1064, 28.8512) -> (51.1556, 32.2301)
  line L770 (51.1556, 25.4724) -> (53.1064, 28.8512)
  line L771 (47.254, 25.4724) -> (51.1556, 25.4724)
  line L772 (45.3032, 28.8512) -> (47.254, 25.4724)
  line L773 (46.215, 24.8725) -> (44.2642, 28.2514)
  line L774 (44.2642, 21.4936) -> (46.215, 24.8725)
  line L775 (40.3626, 21.4936) -> (44.2642, 21.4936)
  line L776 (44.2642, 28.2514) -> (40.3626, 28.2514)
  line L777 (40.3626, 28.2514) -> (38.4118, 24.8725)
  line L778 (38.4118, 24.8725) -> (40.3626, 21.4936)
  line L779 (65.2604, 32.2301) -> (61.3588, 32.2301)
  line L780 (61.3588, 32.2301) -> (59.408, 28.8512)
  line L781 (67.2112, 28.8512) -> (65.2604, 32.2301)
  line L782 (65.2604, 25.4724) -> (67.2112, 28.8512)
  line L783 (61.3588, 25.4724) -> (65.2604, 25.4724)
  line L784 (59.408, 28.8512) -> (61.3588, 25.4724)
  line L785 (60.3198, 24.8725) -> (58.369, 28.2514)
  line L786 (58.369, 21.4936) -> (60.3198, 24.8725)
  line L787 (54.4674, 21.4936) -> (58.369, 21.4936)
  line L788 (58.369, 28.2514) -> (54.4674, 28.2514)
  line L789 (54.4674, 28.2514) -> (52.5166, 24.8725)
  line L790 (52.5166, 24.8725) -> (54.4674, 21.4936)
  line L791 (79.3652, 32.2301) -> (75.4636, 32.2301)
  line L792 (75.4636, 32.2301) -> (73.5128, 28.8512)
  line L793 (81.316, 28.8512) -> (79.3652, 32.2301)
  line L794 (79.3652, 25.4724) -> (81.316, 28.8512)
  line L795 (75.4636, 25.4724) -> (79.3652, 25.4724)
  line L796 (73.5128, 28.8512) -> (75.4636, 25.4724)
  line L797 (74.4246, 24.8725) -> (72.4738, 28.2514)
  line L798 (72.4738, 21.4936) -> (74.4246, 24.8725)
  line L799 (68.5722, 21.4936) -> (72.4738, 21.4936)
  line L800 (72.4738, 28.2514) -> (68.5722, 28.2514)
  line L801 (68.5722, 28.2514) -> (66.6214, 24.8725)
  line L802 (66.6214, 24.8725) -> (68.5722, 21.4936)
  line L803 (76.4154, 30.2181) -> (-71.524, 30.2181)
  line L804 (-71.524, 30.2181) -> (-71.524, -16.6044)
  line L805 (-71.524, -16.6044) -> (76.4154, -16.6044)
  line L806 (76.4154, -16.6044) -> (76.4154, 30.2181)
  point P0 (-0.001, 1)
  dimension "d67" = 0.001
  dimension "d68" = 1
  dimension "d69" = 3.9016
  dimension "d72" = 7.9575
  dimension "d73" = 0
  dimension "d74" = 1.2
  dimension "d77" = 14.1048
  dimension "d78" = 7.9575
  dimension "d79" = 1.2
  dimension "d80" = 5.1016
  dimension "d82" = 1.2
  constraint horizontal L0
  constraint vertical L1
  constraint horizontal L2
  constraint vertical L3
  constraint coincident L0.start L3.end
  constraint coincident P0 L1.end
  constraint midpoint L8 L10.end
  constraint midpoint L6 L11.end
  constraint horizontal L9
  constraint perpendicular L8 L18
  constraint midpoint L9 L43.start
  constraint perpendicular L27 L43
  constraint horizontal L44
  constraint perpendicular L44 L45
  constraint perpendicular L45 L82
  constraint horizontal L803
  constraint vertical L804
  constraint horizontal L805
  constraint vertical L806
  measures "d67" distance of L0.start L0.end
  measures "d68" distance of L0.start L2.end
  measures "d69" distance of L4.start P0
  measures "d74" distance of L10.end L18.end
  measures "d79" distance of L43.start L43.end
  measures "d80" distance of L7.end L44.end
  measures "d82" distance of L44.end L82.end
sketch "Side Panel" plane through (0, 0, 0) normal (1, 0, 0) x (0, 1, 0)
  line L0 (-64.9, 0) -> (64.9, 0)
  line L1 (64.9, 0) -> (64.9, 25.05)
  line L2 (64.9, 25.05) -> (-64.9, 25.05)
  line L3 (-64.9, 25.05) -> (-64.9, 0)
  line L4 (-62.5, 2.4) -> (62.5, 2.4)
  line L5 (62.5, 2.4) -> (62.5, 22.65)
  line L6 (62.5, 22.65) -> (-62.5, 22.65)
  line L7 (-62.5, 22.65) -> (-62.5, 2.4)
  line L8 (60.1, 2.5) -> (62.5, 2.5)
  line L9 (62.5, 25.05) -> (-62.5, 25.05)
  line L10 (-60.1, 0) -> (60.1, 0)
  line L11 (60.1, 0) -> (60.1, 2.5)
  line L12 (62.5, 2.5) -> (62.5, 25.05)
  line L13 (-62.5, 25.05) -> (-62.5, 2.5)
  line L14 (-62.5, 2.5) -> (-60.1, 2.5)
  line L15 (-60.1, 2.5) -> (-60.1, 0)
  dimension "d83" = -2.4
extrude "Extrude9" add sketch "Side Panel" against normal up to surface (4 mm away) from surface at 78.5 separate body contours L4 L5 L6 L7 L8 L11 L12 L13 L14 L15 | L4 L7 L14 L15 | L4 L5 L8 L11 makes body 5
combine "Combine1" operation cut target body 1 tool bodies 5 keep tools
extrude "Extrude10" add sketch "Side Panel" along normal blind 2.4 from surface at 6 separate body contours L4 L5 L6 L7 L8 L11 L12 L13 L14 L15 makes body 6
combine "Combine2" operation cut target body 1 tool bodies 6 keep tools
extrude "Extrude11" cut sketch "Hex Side" along normal blind 80 contours L25 L26 L28 L52 L53 L55 L56 L57 L64 L65 L66 L67 L76 L77 L78 L79 L89 L90 L92 L93 L94 L101 L102 L104 L105 L106 L113 L114 L116 L117 L118 L125 L126 L128 L129 L130 L137 L138 L140 L141 L142 L149 L150 L152 L153 L154 L161 L162 L164 L165 L166 L173 L174 L176 L177 L178 L179 L180 L183 L184 L185 L186 L188 L189 L190 L287 L288 L291 L292 L395 L396 L399 L400 L413 L414 L415 L416 L527 L528 L531 L532 L545 L546 L547 L548 L659 L660 L663 L664 L672 L673 L674 L675 L676 L677 L678 L679 L680 L684 L685 L686 L687 L688 L696 L697 L698 L699 L700 L708 L709 L710 L711 L712 L720 L721 L722 L723 L724 L732 L733 L734 L735 L736 L744 L745 L746 L747 L748 L756 L757 L758 L759 L760 L768 L769 L770 L771 L772 L780 L781 L782 L783 L784 L792 L795 L796 L803 L804 L805 L806 keep common part bodies 5 6
combine "Combine3" operation add target body 1 tool bodies 4 5 6
chamfer "Chamfer3" distance 0.4 angle 45 16 edges at (6, 0, 0) (42.25, 64.9, 0) (6, 64.9, 12.525) (78.5, 0, 0) (78.5, -64.9, 12.525) (42.25, -64.9, 0) (62.8, -64.9, 15.725) (64, -64.9, 6.4) (65.2, -64.9, 4.45) (69.85, -64.9, 2.5) (74.5, -64.9, 13.775) (6, -64.9, 12.525) (78.5, 64.9, 12.525) (16.5, 64.9, 21.025) (36.5, 64.9, 17) (56.5, 64.9, 21.025) on bodies 1
equation "d5 = d4 - 2.4 mm"
equation "d80 = 1.2 mm + 3.9016 mm"
named bodies: "[a]BTT_MMB_case_top"
